bearing_1.5_4_2 v1 (Autodesk Fusion 360 design; units mm, degrees)
Autodesk Fusion 360 part; units mm, degrees
sketch "スケッチ1" plane through (0, 0, 0) normal (0, 0, 1) x (1, 0, 0)
  circle A0 centre (0, 0) radius 2
  circle A1 centre (0, 0) radius 1.7
  circle A2 centre (0, 0) radius 1.05
  circle A3 centre (0, 0) radius 0.75
  dimension "d1" = 4
  dimension "d2" = 1.5
  dimension "d3" = 2.1
  dimension "d4" = 3.4
  measures "d1" diameter of A0
  measures "d2" diameter of A3
  measures "d3" diameter of A2
  measures "d4" diameter of A1
extrude "押し出し1" add sketch "スケッチ1" along normal blind 2 contours A0 makes body 1
extrude "押し出し2" add sketch "スケッチ1" along normal blind 1.6 from surface at 0.2 separate body contours A1 makes body 2
extrude "押し出し1'" add sketch "スケッチ1" along normal blind 2 separate body contours A2 makes body 3 in component "Component"
component "Component" placed x (1, 0, 0) y (0, 1, 0) z (0, 0, 1) at (0, 0, 0)
